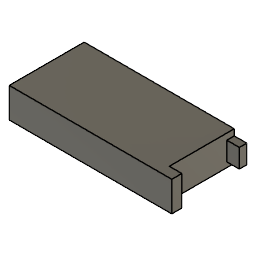
battery (Autodesk Fusion 360 design; units mm, degrees)
Autodesk Fusion 360 part; units mm, degrees
sketch "Sketch1" plane through (0, 0, 0) normal (0, 0, 1) x (1, 0, 0)
  line L0 (0, 0) -> (60, 0)
  line L1 (60, 0) -> (60, 30)
  line L2 (60, 30) -> (0, 30)
  line L3 (0, 30) -> (0, 0)
  dimension "d1" = 30
  dimension "d2" = 60
  constraint horizontal L0
  constraint vertical L1
  constraint horizontal L2
  constraint vertical L3
  constraint coincident L0.start L3.end
  measures "d1" distance of L0.start L2.end
  measures "d2" distance of L0.start L0.end
extrude "Extrude1" add sketch "Sketch1" along normal blind 12
sketch "Sketch2" plane through (60, 0, 0) normal (1, 0, 0) x (0, 1, 0)
  line L0 (0, 0) -> (30, 0)
  line L1 (30, 0) -> (30, 12)
  line L2 (30, 12) -> (0, 12)
  line L3 (0, 12) -> (0, 0)
  line L4 (0, 12) -> (4, 12)
  line L5 (4, 12) -> (4, 0)
  line L6 (4, 0) -> (0, 0)
  line L7 (0, 0) -> (0, 12)
  line L8 (30, 9.5242) -> (27, 9.5242)
  line L9 (27, 9.5242) -> (27, 2)
  line L10 (27, 2) -> (30, 2)
  line L11 (30, 2) -> (30, 9.5242)
  constraint horizontal L4
  constraint vertical L5
  constraint horizontal L6
  constraint vertical L7
  constraint coincident L0 L5.end
  constraint coincident L2.end L3.start
  constraint horizontal L8
  constraint vertical L9
  constraint horizontal L10
  constraint vertical L11
  constraint coincident L1 L8.start
extrude "Extrude2" add sketch "Sketch2" along normal blind 5 contours L0 L2 L3 L4 L5 L6 L7 | L1 L8 L9 L10 L11
